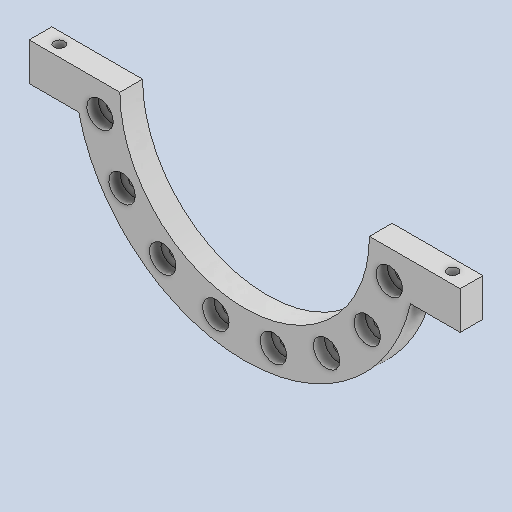
# Autodesk Inventor part: ДМФ 091 Постель НОС v2.0
Saved by Autodesk Inventor 2025 (Build 290162010, 162A)
## iProperties
Created: 2024-04-28
Part Number: ДМФ 091 Постель НОС v2.0
Material: Generic
Document SubType Name: Sheet Metal
Designer: admin
Density: 1 g/cm^3
Appearance: Default
Stock Number: Постель_Нос
Flat Pattern Width: 22.5 cm
Flat Pattern Length: 57 cm
Flat Pattern Area: 1282.5 cm^2
Sheet Metal Rule: Default
Sheet Metal Width: 225,000 mm
Sheet Metal Length: 570,000 mm
Sheet Metal Area: 128250,000 mm^2
Author: pokla
Autodesk Inventor part; units mm, degrees
ref_plane "YZ Plane" through (0, 0, 0) normal (1, 0, 0) x (0, 1, 0)
ref_plane "XZ Plane" through (0, 0, 0) normal (0, 1, 0) x (-1, 0, 0)
ref_plane "XY Plane" through (0, 0, 0) normal (0, 0, 1) x (1, 0, 0)
sketch "Sketch1" plane through (0, 0, 0) normal (0, 0, 1) x (1, 0, 0)
  circle A0 centre (0, 0) radius 195 construction
  line L0 (0, 195) -> (0, 225) construction
  line L1 (0, 195) -> (0, 165) construction
  circle A1 centre (0, 0) radius 165
  circle A2 centre (0, 0) radius 225
  line L2 (-165, 0) -> (-165, 80)
  line L3 (-165, 80) -> (-225, 80)
  line L4 (-225, 80) -> (-225, 0)
  line L5 (165, 0) -> (165, 80)
  line L6 (165, 80) -> (225, 80)
  line L7 (225, 80) -> (225, 0)
  line L8 (-225, 0) -> (-165, 0)
  line L9 (165, 0) -> (225, 0)
  line L10 (-225, 0) -> (-285, 0)
  line L11 (-285, 0) -> (-285, -50)
  line L12 (-285, -50) -> (-219.3741, -50)
  line L13 (225, 0) -> (285, 0)
  line L14 (285, 0) -> (285, -50)
  line L15 (285, -50) -> (219.3741, -50)
  dimension "d13" = 390
  dimension "d26" = 80
  dimension "d36" = 60
  dimension "d40" = 60
  dimension "d41" = 50
  constraints: 32 end point, 8 point on circle, 7 perpendicular, 4 equal length, 4 horizontal, 4 tangent, 4 vertical, 3 coincident, 2 centre point, 1 line through centre, 1 point on line, 1 vertical alignment, 2 other
  measures "d26" distance of L2.start L2.end
  measures "d36" distance of L1.end L0.end
  measures "d40" distance of L4.end L10.end
  measures "d41" distance of L10.end L11.end
extrude "Extrusion1" add sketch "Sketch1" against normal blind 30 contours L9 A2 L8 A1 | L13 L14 L15 A2 | A2 L12 L11 L10
sketch "Sketch4" plane through (0, 0, 0) normal (0, 0, 1) x (1, 0, 0)
  circle A0 centre (38.0426, -191.2531) radius 6.5
  line L0 (0, 0) -> (38.0426, -191.2531) construction
  line L1 (0, 0) -> (0, -276.8337) construction
  dimension "d17" = 13
  dimension "d27" = 195
  dimension "d35" = 11.25
  constraints: 4 end point, 1 centre point, 1 vertical
  measures "d17" diameter of A0
  measures "d27" distance of L0.end L0.start
  measures "d35" angle of L1 L0
extrude "Extrusion4" cut sketch "Sketch4" against normal through all
sketch "Sketch5" plane through (0, 0, 0) normal (0, 0, 1) x (1, 0, 0)
  circle A0 centre (38.0426, -191.2531) radius 6.5 projected
  circle A1 centre (38.0426, -191.2531) radius 17.5
  point P0 (0, 0)
  dimension "d23" = 35
  constraints: 1 centre point, 1 coincident
  measures "d23" diameter of A1
extrude "Extrusion5" cut sketch "Sketch5" against normal blind 15
pattern_circular "Circular Pattern3" count 8 over 157.5 about axis through (0, 0, 0) along (0, 0, -1) of "Extrusion4", "Extrusion5" both ways yes
sketch "Sketch7" plane through (-285, 0, 0) normal (0, 1, 0) x (1, 0, 0)
  circle A0 centre (25, 15) radius 7
  line L0 (0, 0) -> (0, 30) projected
  point P0 (285, 0)
  point P1 (0, 15)
  dimension "d42" = 14
  dimension "d43" = 25
  constraints: 1 centre point, 1 horizontal alignment, 1 midpoint
  measures "d42" diameter of A0
  measures "d43" distance from line of L0 A0.centre
extrude "Extrusion7" cut sketch "Sketch7" against normal through all
mirror "Mirror1" about plane through (0, 0, 0) normal (1, 0, 0) of "Extrusion7"
equation "\"d13\" = Шпил_пласт_НОС_диам_центров"
equation "\"d40\" = d36"
equation "\"d27\" = 0.5 * Шпил_пласт_НОС_диам_центров"
equation "\"BendReliefDepth\" = 0.5 * Thickness"
equation "\"Шпил_пласт_НОС_диам_центров\" = 390"
equation "\"Thickness\" = 30"
body "Solid1"
